Autodesk Inventor part; units mm, degrees
(part 2 of 2)
  spline S169 degree 2 poles (5.3322, -2.7566) (5.3322, -3.0199) (5.6199, -3.2185) (5.8995, -3.2185) knots 0 0 0 1 2 2 2
  spline S170 degree 2 poles (5.8995, -3.2185) (6.0535, -3.2185) (6.3776, -3.0767) (6.5073, -2.9511) knots 0 0 0 1 2 2 2
  line L157 (9.9433, 1.0643) -> (9.8055, -2.4932)
  line L158 (9.8055, -2.4932) -> (8.7439, -2.4932)
  line L159 (8.7439, -2.4932) -> (8.6061, 1.0643)
  line L160 (8.6061, 1.0643) -> (9.9433, 1.0643)
  line L161 (9.9352, -3.9357) -> (8.6142, -3.9357)
  line L162 (8.6142, -3.9357) -> (8.6142, -3.0483)
  line L163 (8.6142, -3.0483) -> (9.9352, -3.0483)
  line L164 (9.9352, -3.0483) -> (9.9352, -3.9357)
  line L165 (-16.0555, -12.168) -> (-14.3659, -7.168)
  line L166 (-14.3659, -7.168) -> (-12.9964, -7.168)
  line L167 (-12.9964, -7.168) -> (-11.3067, -12.168)
  line L168 (-11.3067, -12.168) -> (-12.5993, -12.168)
  line L169 (-12.5993, -12.168) -> (-12.9113, -11.147)
  line L170 (-12.9113, -11.147) -> (-14.4834, -11.147)
  line L171 (-14.4834, -11.147) -> (-14.7994, -12.168)
  line L172 (-14.7994, -12.168) -> (-16.0555, -12.168)
  line L173 (-13.1868, -10.2393) -> (-13.6973, -8.5862)
  line L174 (-13.6973, -8.5862) -> (-14.2119, -10.2393)
  line L175 (-14.2119, -10.2393) -> (-13.1868, -10.2393)
  spline S171 degree 2 poles (-8.7986, -11.7669) (-8.9202, -11.8682) (-9.1106, -12.0303) (-9.2727, -12.1113) knots 0 0 0 1 2 2 2
  spline S172 degree 2 poles (-9.2727, -12.1113) (-9.4307, -12.1883) (-9.7306, -12.2693) (-9.998, -12.2693) knots 0 0 0 1 2 2 2
  spline S173 degree 2 poles (-9.998, -12.2693) (-10.5004, -12.2693) (-11.1609, -11.5967) (-11.1609, -11.0862) knots 0 0 0 1 2 2 2
  spline S174 degree 2 poles (-11.1609, -11.0862) (-11.1609, -10.6688) (-10.8246, -10.1502) (-10.5085, -10.0003) knots 0 0 0 1 2 2 2
  spline S175 degree 2 poles (-10.5085, -10.0003) (-10.1884, -9.8463) (-9.3011, -9.7248) (-8.7905, -9.6923) knots 0 0 0 1 2 2 2
  line L176 (-8.7905, -9.6923) -> (-8.7905, -9.6721)
  spline S176 degree 2 poles (-8.7905, -9.6721) (-8.7905, -9.3601) (-9.2524, -9.121) (-9.7144, -9.121) knots 0 0 0 1 2 2 2
  spline S177 degree 2 poles (-9.7144, -9.121) (-9.921, -9.121) (-10.4802, -9.2709) (-10.7435, -9.3884) knots 0 0 0 1 2 2 2
  line L177 (-10.7435, -9.3884) -> (-10.8448, -9.3884)
  line L178 (-10.8448, -9.3884) -> (-10.8448, -8.4768)
  spline S178 degree 2 poles (-10.8448, -8.4768) (-10.6706, -8.4282) (-9.8926, -8.2904) (-9.4956, -8.2904) knots 0 0 0 1 2 2 2
  spline S179 degree 2 poles (-9.4956, -8.2904) (-8.5231, -8.2904) (-7.6317, -8.9387) (-7.6317, -9.6032) knots 0 0 0 1 2 2 2
  line L179 (-7.6317, -9.6032) -> (-7.6317, -12.168)
  line L180 (-7.6317, -12.168) -> (-8.7986, -12.168)
  line L181 (-8.7986, -12.168) -> (-8.7986, -11.7669)
  line L182 (-8.7986, -11.1834) -> (-8.7986, -10.4014)
  spline S180 degree 2 poles (-8.7986, -10.4014) (-9.0985, -10.4298) (-9.4672, -10.4743) (-9.6455, -10.5392) knots 0 0 0 1 2 2 2
  spline S181 degree 2 poles (-9.6455, -10.5392) (-9.8035, -10.5918) (-9.9737, -10.8107) (-9.9737, -10.9889) knots 0 0 0 1 2 2 2
  spline S182 degree 2 poles (-9.9737, -10.9889) (-9.9737, -11.2523) (-9.686, -11.4508) (-9.4064, -11.4508) knots 0 0 0 1 2 2 2
  spline S183 degree 2 poles (-9.4064, -11.4508) (-9.2524, -11.4508) (-8.9283, -11.309) (-8.7986, -11.1834) knots 0 0 0 1 2 2 2
  line L183 (-2.2589, -12.168) -> (-2.2589, -10.2839)
  spline S184 degree 2 poles (-2.2589, -10.2839) (-2.2589, -10.0043) (-2.2792, -9.6235) (-2.3278, -9.5019) knots 0 0 0 1 2 2 2
  spline S185 degree 2 poles (-2.3278, -9.5019) (-2.3805, -9.3803) (-2.5912, -9.2709) (-2.7816, -9.2709) knots 0 0 0 1 2 2 2
  spline S186 degree 2 poles (-2.7816, -9.2709) (-2.9153, -9.2709) (-3.1747, -9.3884) (-3.3286, -9.4978) knots 0 0 0 1 2 2 2
  line L184 (-3.3286, -9.4978) -> (-3.3286, -12.168)
  line L185 (-3.3286, -12.168) -> (-4.5118, -12.168)
  line L186 (-4.5118, -12.168) -> (-4.5118, -10.2839)
  spline S187 degree 2 poles (-4.5118, -10.2839) (-4.5118, -10.0084) (-4.5361, -9.6235) (-4.5847, -9.5019) knots 0 0 0 1 2 2 2
  spline S188 degree 2 poles (-4.5847, -9.5019) (-4.6374, -9.3803) (-4.8481, -9.2709) (-5.0385, -9.2709) knots 0 0 0 1 2 2 2
  spline S189 degree 2 poles (-5.0385, -9.2709) (-5.1803, -9.2709) (-5.4599, -9.4047) (-5.5896, -9.4978) knots 0 0 0 1 2 2 2
  line L187 (-5.5896, -9.4978) -> (-5.5896, -12.168)
  line L188 (-5.5896, -12.168) -> (-6.7646, -12.168)
  line L189 (-6.7646, -12.168) -> (-6.7646, -8.3957)
  line L190 (-6.7646, -8.3957) -> (-5.5896, -8.3957)
  line L191 (-5.5896, -8.3957) -> (-5.5896, -8.8131)
  spline S190 degree 2 poles (-5.5896, -8.8131) (-5.3019, -8.57) (-4.7873, -8.2944) (-4.4672, -8.2944) knots 0 0 0 1 2 2 2
  spline S191 degree 2 poles (-4.4672, -8.2944) (-4.1228, -8.2944) (-3.596, -8.6226) (-3.4583, -8.9508) knots 0 0 0 1 2 2 2
  spline S192 degree 2 poles (-3.4583, -8.9508) (-3.122, -8.6348) (-2.5223, -8.2944) (-2.2144, -8.2944) knots 0 0 0 1 2 2 2
  spline S193 degree 2 poles (-2.2144, -8.2944) (-1.951, -8.2944) (-1.5336, -8.4606) (-1.3918, -8.6307) knots 0 0 0 1 2 2 2
  spline S194 degree 2 poles (-1.3918, -8.6307) (-1.2338, -8.8131) (-1.0758, -9.3115) (-1.0758, -9.7126) knots 0 0 0 1 2 2 2
  line L192 (-1.0758, -9.7126) -> (-1.0758, -12.168)
  line L193 (-1.0758, -12.168) -> (-2.2589, -12.168)
  line L194 (0.9704, -12.168) -> (-0.2046, -12.168)
  line L195 (-0.2046, -12.168) -> (-0.2046, -8.3957)
  line L196 (-0.2046, -8.3957) -> (0.9704, -8.3957)
  line L197 (0.9704, -8.3957) -> (0.9704, -12.168)
  line L198 (1.0069, -7.8568) -> (-0.2371, -7.8568)
  line L199 (-0.2371, -7.8568) -> (-0.2371, -6.9411)
  line L200 (-0.2371, -6.9411) -> (1.0069, -6.9411)
  line L201 (1.0069, -6.9411) -> (1.0069, -7.8568)
  line L202 (3.045, -12.168) -> (1.8699, -12.168)
  line L203 (1.8699, -12.168) -> (1.8699, -8.3957)
  line L204 (1.8699, -8.3957) -> (3.045, -8.3957)
  line L205 (3.045, -8.3957) -> (3.045, -12.168)
  line L206 (3.0814, -7.8568) -> (1.8375, -7.8568)
  line L207 (1.8375, -7.8568) -> (1.8375, -6.9411)
  line L208 (1.8375, -6.9411) -> (3.0814, -6.9411)
  line L209 (3.0814, -6.9411) -> (3.0814, -7.8568)
  line L210 (7.4736, -12.168) -> (6.2905, -12.168)
  line L211 (6.2905, -12.168) -> (6.2905, -10.3001)
  spline S195 degree 2 poles (6.2905, -10.3001) (6.2905, -10.0692) (6.254, -9.6154) (6.2054, -9.51) knots 0 0 0 1 2 2 2
  spline S196 degree 2 poles (6.2054, -9.51) (6.1446, -9.3803) (5.9177, -9.2709) (5.7232, -9.2709) knots 0 0 0 1 2 2 2
  spline S197 degree 2 poles (5.7232, -9.2709) (5.5814, -9.2709) (5.2856, -9.3803) (5.1195, -9.4978) knots 0 0 0 1 2 2 2
  line L212 (5.1195, -9.4978) -> (5.1195, -12.168)
  line L213 (5.1195, -12.168) -> (3.9445, -12.168)
  line L214 (3.9445, -12.168) -> (3.9445, -8.3957)
  line L215 (3.9445, -8.3957) -> (5.1195, -8.3957)
  line L216 (5.1195, -8.3957) -> (5.1195, -8.8131)
  spline S198 degree 2 poles (5.1195, -8.8131) (5.4072, -8.57) (5.9542, -8.2944) (6.2864, -8.2944) knots 0 0 0 1 2 2 2
  spline S199 degree 2 poles (6.2864, -8.2944) (6.8618, -8.2944) (7.4736, -9.0238) (7.4736, -9.7126) knots 0 0 0 1 2 2 2
  line L217 (7.4736, -9.7126) -> (7.4736, -12.168)
  line L218 (11.7524, -12.168) -> (10.5652, -12.168)
  line L219 (10.5652, -12.168) -> (10.5652, -10.8471)
  line L220 (10.5652, -10.8471) -> (11.7524, -10.8471)
  line L221 (11.7524, -10.8471) -> (11.7524, -12.168)
  line L222 (11.7524, -9.7166) -> (10.5652, -9.7166)
  line L223 (10.5652, -9.7166) -> (10.5652, -8.3957)
  line L224 (10.5652, -8.3957) -> (11.7524, -8.3957)
  line L225 (11.7524, -8.3957) -> (11.7524, -9.7166)
  spline S200 degree 2 poles (15.1519, -10.2474) (15.1519, -10.7539) (14.9736, -11.6899) (14.8156, -12.0789) knots 0 0 0 1 2 2 2
  spline S201 degree 2 poles (14.8156, -12.0789) (14.6495, -12.4922) (14.1835, -13.2094) (13.8999, -13.5497) knots 0 0 0 1 2 2 2
  line L226 (13.8999, -13.5497) -> (12.6681, -13.5497)
  line L227 (12.6681, -13.5497) -> (12.6681, -13.4525)
  spline S202 degree 2 poles (12.6681, -13.4525) (12.9356, -13.2134) (13.4461, -12.5692) (13.6446, -12.1721) knots 0 0 0 1 2 2 2
  spline S203 degree 2 poles (13.6446, -12.1721) (13.8553, -11.7547) (14.0984, -10.8228) (14.0984, -10.2474) knots 0 0 0 1 2 2 2
  spline S204 degree 2 poles (14.0984, -10.2474) (14.0984, -9.6964) (13.8472, -8.7239) (13.6446, -8.3228) knots 0 0 0 1 2 2 2
  spline S205 degree 2 poles (13.6446, -8.3228) (13.4339, -7.9095) (12.9396, -7.2855) (12.6681, -7.0424) knots 0 0 0 1 2 2 2
  line L228 (12.6681, -7.0424) -> (12.6681, -6.9452)
  line L229 (12.6681, -6.9452) -> (13.8999, -6.9452)
  spline S206 degree 2 poles (13.8999, -6.9452) (14.1916, -7.2936) (14.6576, -8.0149) (14.8197, -8.4201) knots 0 0 0 1 2 2 2
  spline S207 degree 2 poles (14.8197, -8.4201) (14.9655, -8.7928) (15.1519, -9.6923) (15.1519, -10.2474) knots 0 0 0 1 2 2 2
  point P0 (0, 0)
  constraints: 2 other
extrude "Extrusion14" add sketch "Sketch19" along normal blind 3
body "Solid1"
